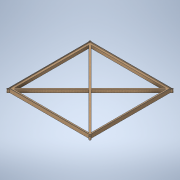
# Autodesk Inventor part: base de calibração
Saved by Autodesk Inventor 2022 (Build 260153000, 153)
## iProperties
Created: 2022-02-16
Part Number: base de calibração
Material: MDF - Chapa de fibra de média densidade
Document SubType Name: Modeling
Designer: mathe
Density: 0.8 g/cm^3
Appearance: Papelão - Corrugado
Mass: 397.943 g
Surface Area: 1633.83 cm^2
Volume: 497.429 cm^3
Author: mathe
Autodesk Inventor part; units mm, degrees
ref_plane "YZ Plane" through (0, 0, 0) normal (1, 0, 0) x (0, 1, 0)
ref_plane "XZ Plane" through (0, 0, 0) normal (0, 1, 0) x (-1, 0, 0)
ref_plane "XY Plane" through (0, 0, 0) normal (0, 0, 1) x (1, 0, 0)
sketch "Esboço1" plane through (0, 0, 0) normal (0, 0, 1) x (1, 0, 0)
  line L0 (7.0711, 0) -> (422.9289, 0)
  line L1 (430, 7.0711) -> (430, 422.9289)
  line L2 (422.9289, 430) -> (7.0711, 430)
  line L3 (0, 422.9289) -> (0, 7.0711)
  line L4 (17.0711, 420) -> (412.9289, 420)
  line L5 (420, 412.9289) -> (420, 17.0711)
  line L6 (412.9289, 10) -> (17.0711, 10)
  line L7 (10, 17.0711) -> (10, 412.9289)
  line L8 (420, 17.0711) -> (222.0711, 215)
  line L9 (215, 222.0711) -> (17.0711, 420)
  line L10 (412.9289, 10) -> (215, 207.9289)
  line L11 (207.9289, 215) -> (10, 412.9289)
  line L12 (10, 17.0711) -> (207.9289, 215)
  line L13 (215, 222.0711) -> (412.9289, 420)
  line L14 (17.0711, 10) -> (215, 207.9289)
  line L15 (222.0711, 215) -> (420, 412.9289)
  line L16 (425.0292, 432.1003) -> (430.6066, 437.6777)
  line L17 (437.6777, 437.6777) -> (437.6777, 437.6777)
  line L18 (437.6777, 430.6066) -> (432.1421, 425.0711)
  line L19 (-2.1003, 425.0292) -> (-7.6777, 430.6066)
  line L20 (-7.6777, 437.6777) -> (-7.6777, 437.6777)
  line L21 (-0.6066, 437.6777) -> (4.9708, 432.1003)
  line L22 (4.9289, -2.1421) -> (-0.6066, -7.6777)
  line L23 (-7.6777, -7.6777) -> (-7.6777, -7.6777)
  line L24 (-7.6777, -0.6066) -> (-2.1003, 4.9708)
  line L25 (425.0711, -2.1421) -> (430.6066, -7.6777)
  line L26 (437.6777, -7.6777) -> (437.6777, -7.6777)
  line L27 (437.6777, -0.6066) -> (432.1421, 4.9289)
  arc A0 (437.6777, 430.6066) -> (437.6777, 437.6777) centre (434.1421, 434.1421) ccw
  arc A1 (437.6777, 437.6777) -> (430.6066, 437.6777) centre (434.1421, 434.1421) ccw
  arc A2 (-0.6066, 437.6777) -> (-7.6777, 437.6777) centre (-4.1421, 434.1421) ccw
  arc A3 (-7.6777, 437.6777) -> (-7.6777, 430.6066) centre (-4.1421, 434.1421) ccw
  arc A4 (-7.6777, -0.6066) -> (-7.6777, -7.6777) centre (-4.1421, -4.1421) ccw
  arc A5 (-7.6777, -7.6777) -> (-0.6066, -7.6777) centre (-4.1421, -4.1421) ccw
  arc A6 (430.6066, -7.6777) -> (437.6777, -7.6777) centre (434.1421, -4.1421) ccw
  arc A7 (437.6777, -7.6777) -> (437.6777, -0.6066) centre (434.1421, -4.1421) ccw
  circle A8 centre (-4.1421, 434.1421) radius 2
  circle A9 centre (434.1421, 434.1421) radius 2
  circle A10 centre (434.1421, -4.1421) radius 2
  circle A11 centre (-4.1421, -4.1421) radius 2
  line L28 (432.1421, 432.1003) -> (-2.1003, 432.1003)
  line L29 (-2.1003, 432.1003) -> (-2.1003, -2.1421)
  line L30 (-2.1003, -2.1421) -> (432.1421, -2.1421)
  line L31 (432.1421, -2.1421) -> (432.1421, 432.1003)
  line L32 (0, 0) -> (430, 0)
  line L33 (430, 0) -> (430, 430)
  line L34 (430, 430) -> (0, 430)
  line L35 (0, 430) -> (0, 0)
  point P0 (-7.6777, -7.6777)
  dimension "d2" = 10
  dimension "d11" = 5
  dimension "d12" = 4
  dimension "d13" = 4
  dimension "d14" = 4
  dimension "d15" = 4
  constraints: 72 end point, 16 point on circle, 16 tangent, 12 centre point, 12 parallel, 8 point on line, 7 equal radius, 4 coincident, 4 perpendicular, 3 horizontal
  measures "d2" distance between parallel lines of L2 L4
  measures "d11" radius of A0
  measures "d12" diameter of A8
  measures "d13" diameter of A9
  measures "d14" diameter of A10
  measures "d15" diameter of A11
extrude "Extrusão2" add sketch "Esboço1" along normal blind 15 contours L32 L35 L3 L34 L2 L33 L1 L0 | L16 A1 A0 L18 L31 L28 | L28 L29 L19 A3 A2 L21 | L27 A7 A6 L25 L30 L31 | L29 L30 L22 A5 A4 L24
extrude "Extrusão3" add sketch "Esboço1" along normal blind 15 and the other way blind 4 contours L28 L31 L30 L29
